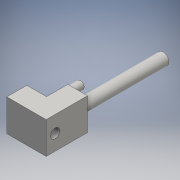
# Autodesk Inventor part: 240503_3Dsketch01
Saved by Autodesk Inventor 2016 (Build 200138000, 138)
## iProperties
Created: 2024-05-03
Part Number: 240503_3Dsketch01
Material: 일반
Document SubType Name: Modeling
Designer: pc
Density: 1 g/cm^3
Appearance: 기본값
Author: pc
Autodesk Inventor part; units mm, degrees
ref_plane "YZ Plane" through (0, 0, 0) normal (1, 0, 0) x (0, 1, 0)
ref_plane "XZ Plane" through (0, 0, 0) normal (0, 1, 0) x (-1, 0, 0)
ref_plane "XY Plane" through (0, 0, 0) normal (0, 0, 1) x (1, 0, 0)
sketch "스케치1" plane through (0, 0, 0) normal (0, 0, 1) x (1, 0, 0)
  line L0 (36.9529, -18.7887) -> (-36.9529, -18.7887)
  line L1 (-36.9529, -18.7887) -> (-36.9529, 18.7887)
  line L2 (-36.9529, 18.7887) -> (36.9529, 18.7887)
  line L3 (36.9529, 18.7887) -> (36.9529, -18.7887)
  line L4 (36.9529, -18.7887) -> (-36.9529, 18.7887) construction
  line L5 (-36.9529, -18.7887) -> (36.9529, 18.7887) construction
  point P0 (0, 0)
  constraints: 12 end point, 2 midpoint, 2 parallel, 1 horizontal, 1 perpendicular
extrude "돌출1" add sketch "스케치1" along normal blind 60
sketch "스케치2" plane through (-36.9529, 18.7887, 0) normal (0, 1, 0) x (1, 0, 0)
  line L0 (73.9059, 0) -> (73.9059, -60) projected
  line L1 (36.9529, 0) -> (73.9059, 0)
  line L2 (73.9059, 0) -> (73.9059, -60)
  line L3 (73.9059, -60) -> (36.9529, -60)
  line L4 (36.9529, -60) -> (36.9529, 0)
  circle A0 centre (55.4294, -30) radius 7.9669
  constraints: 8 end point, 2 parallel, 1 centre point, 1 horizontal, 1 perpendicular
extrude "돌출2" add sketch "스케치2" along normal blind 40 contours L0 L3 L4 L1 | A0
sketch "스케치3" plane through (-36.9529, 18.7887, 60) normal (0, 1, 0) x (1, 0, 0)
  circle A0 centre (19.9645, 29.7419) radius 7.2214
  point P0 (36.9529, 60)
  constraints: 1 centre point
extrude "돌출3" add sketch "스케치3" along normal blind 80.5
sketch "스케치4" plane through (-36.9529, 58.7887, 0) normal (0, 1, 0) x (1, 0, 0)
  circle A0 centre (55.3783, -30.6807) radius 10.7619
  point P0 (36.9529, 0)
  constraints: 1 centre point
extrude "돌출4" add sketch "스케치4" along normal blind 161
sketch "스케치5" plane through (-36.9529, -18.7887, 0) normal (-1, 0, 0) x (0, 0, 1)
  circle A0 centre (29.4129, 16.6757) radius 8.7461
  point P0 (0, 18.7887)
  constraints: 1 centre point
extrude "돌출5" cut sketch "스케치5" against normal blind 80.5
